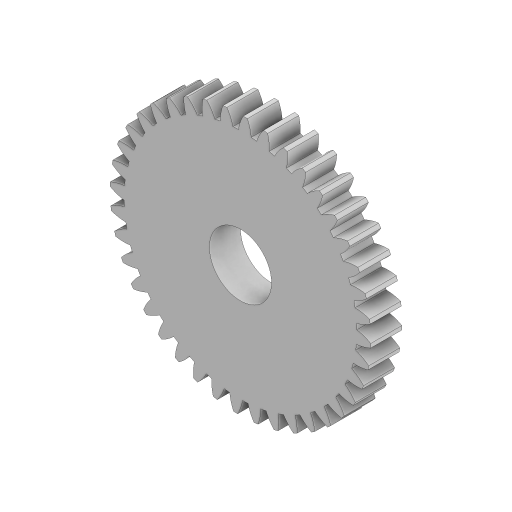
# Autodesk Inventor part: ENGRANAJE PARA RODILLO CONDUCIDO
Saved by Autodesk Inventor 2024 (Build 280153000, 153)
## iProperties
Created: 2024-06-28
Part Number: ENGRANAJE PARA RODILLO CONDUCIDO
Material: Generic
Document SubType Name: Modeling
Designer: Jhuliams
Density: 1 g/cm^3
Appearance: Default
Author: Jhuliams
Autodesk Inventor part; units mm, degrees
ref_plane "YZ Plane" through (0, 0, 0) normal (1, 0, 0) x (0, 1, 0)
ref_plane "XZ Plane" through (0, 0, 0) normal (0, 1, 0) x (-1, 0, 0)
ref_plane "XY Plane" through (0, 0, 0) normal (0, 0, 1) x (1, 0, 0)
sketch "Sketch1" plane through (0, 0, 0) normal (0, 0, 1) x (1, 0, 0)
  arc A0 (41.9411, -2.2239) -> (41.9901, -0.9106) centre (0, 0) ccw
  circle A1 centre (0, 0) radius 37.5
  line L0 (0, 0) -> (54.0602, 0) construction
  line L1 (0, 0) -> (50, 0) construction
  arc A2 (41.9901, -0.9106) -> (37.4943, 0.6513) centre (35.3209, -12.8558) ccw
  arc A3 (37.3413, -3.4461) -> (41.9411, -2.2239) centre (36.1814, 10.1854) ccw
  arc A4 (41.7726, 4.3645) -> (41.6156, 5.6693) centre (0, 0) ccw
  arc A5 (41.6156, 5.6693) -> (36.9308, 6.5087) centre (36.8971, -7.1721) ccw
  arc A6 (37.4207, 2.4377) -> (41.7726, 4.3645) centre (34.1426, 15.72) ccw
  arc A7 (40.5756, 10.8455) -> (40.2164, 12.1096) centre (0, 0) ccw
  arc A8 (40.2164, 12.1096) -> (35.458, 12.2058) centre (37.5648, -1.3118) ccw
  arc A9 (36.5786, 8.2616) -> (40.5756, 10.8455) centre (31.2631, 20.8676) ccw
  arc A10 (38.3794, 17.0593) -> (37.8269, 18.2517) centre (0, 0) ccw
  arc A11 (37.8269, 18.2517) -> (33.112, 17.6024) centre (37.3075, 4.5808) ccw
  arc A12 (34.8359, 13.8821) -> (38.3794, 17.0593) centre (27.6138, 25.5013) ccw
  arc A13 (35.2382, 22.8532) -> (34.506, 23.9445) centre (0, 0) ccw
  arc A14 (34.506, 23.9445) -> (29.9507, 22.5655) centre (36.1316, 10.3606) ccw
  arc A15 (32.2354, 19.1607) -> (35.2382, 22.8532) centre (23.2845, 29.507) ccw
  arc A16 (31.2294, 28.0843) -> (30.3354, 29.0476) centre (0, 0) ccw
  arc A17 (30.3354, 29.0476) -> (26.052, 26.973) centre (34.066, 15.8853) ccw
  arc A18 (28.8411, 23.9675) -> (31.2294, 28.0843) centre (18.3819, 32.7863) ccw
  arc A19 (26.4515, 32.6239) -> (25.4179, 33.4355) centre (0, 0) ccw
  arc A20 (25.4179, 33.4355) -> (21.5117, 30.7164) centre (31.1616, 21.0188) ccw
  arc A21 (24.7367, 28.1842) -> (26.4515, 32.6239) centre (13.0267, 35.2582) ccw
  arc A22 (21.0224, 36.3602) -> (19.8745, 37.0001) centre (0, 0) ccw
  arc A23 (19.8745, 37.0001) -> (16.4418, 33.7034) centre (27.4899, 25.6348) ccw
  arc A24 (20.0231, 31.7068) -> (21.0224, 36.3602) centre (7.3508, 36.8619) ccw
  arc A25 (15.0756, 39.2011) -> (13.8417, 39.6536) centre (0, 0) ccw
  arc A26 (13.8417, 39.6536) -> (10.967, 35.8605) centre (23.1413, 29.6195) ccw
  arc A27 (14.8166, 34.4488) -> (15.0756, 39.2011) centre (1.4938, 37.558) ccw
  arc A28 (8.7575, 41.0768) -> (7.4681, 41.3307) centre (0, 0) ccw
  arc A29 (7.4681, 41.3307) -> (5.2221, 37.1346) centre (18.2229, 32.8749) ccw
  arc A30 (9.2452, 36.3425) -> (8.7575, 41.0768) centre (-4.4, 37.3293) ccw
  arc A31 (2.2239, 41.9411) -> (0.9106, 41.9901) centre (0, 0) ccw
  arc A32 (0.9106, 41.9901) -> (-0.6513, 37.4943) centre (12.8558, 35.3209) ccw
  arc A33 (3.4461, 37.3413) -> (2.2239, 41.9411) centre (-10.1854, 36.1814) ccw
  arc A34 (-4.3645, 41.7726) -> (-5.6693, 41.6156) centre (0, 0) ccw
  arc A35 (-5.6693, 41.6156) -> (-6.5087, 36.9308) centre (7.1721, 36.8971) ccw
  arc A36 (-2.4377, 37.4207) -> (-4.3645, 41.7726) centre (-15.72, 34.1426) ccw
  arc A37 (-10.8455, 40.5756) -> (-12.1096, 40.2164) centre (0, 0) ccw
  arc A38 (-12.1096, 40.2164) -> (-12.2058, 35.458) centre (1.3118, 37.5648) ccw
  arc A39 (-8.2616, 36.5786) -> (-10.8455, 40.5756) centre (-20.8676, 31.2631) ccw
  arc A40 (-17.0593, 38.3794) -> (-18.2517, 37.8269) centre (0, 0) ccw
  arc A41 (-18.2517, 37.8269) -> (-17.6024, 33.112) centre (-4.5808, 37.3075) ccw
  arc A42 (-13.8821, 34.8359) -> (-17.0593, 38.3794) centre (-25.5013, 27.6138) ccw
  arc A43 (-22.8532, 35.2382) -> (-23.9445, 34.506) centre (0, 0) ccw
  arc A44 (-23.9445, 34.506) -> (-22.5655, 29.9507) centre (-10.3606, 36.1316) ccw
  arc A45 (-19.1607, 32.2354) -> (-22.8532, 35.2382) centre (-29.507, 23.2845) ccw
  arc A46 (-28.0843, 31.2294) -> (-29.0476, 30.3354) centre (0, 0) ccw
  arc A47 (-29.0476, 30.3354) -> (-26.973, 26.052) centre (-15.8853, 34.066) ccw
  arc A48 (-23.9675, 28.8411) -> (-28.0843, 31.2294) centre (-32.7863, 18.3819) ccw
  arc A49 (-32.6239, 26.4515) -> (-33.4355, 25.4179) centre (0, 0) ccw
  arc A50 (-33.4355, 25.4179) -> (-30.7164, 21.5117) centre (-21.0188, 31.1616) ccw
  arc A51 (-28.1842, 24.7367) -> (-32.6239, 26.4515) centre (-35.2582, 13.0267) ccw
  arc A52 (-36.3602, 21.0224) -> (-37.0001, 19.8745) centre (0, 0) ccw
  arc A53 (-37.0001, 19.8745) -> (-33.7034, 16.4418) centre (-25.6348, 27.4899) ccw
  arc A54 (-31.7068, 20.0231) -> (-36.3602, 21.0224) centre (-36.8619, 7.3508) ccw
  arc A55 (-39.2011, 15.0756) -> (-39.6536, 13.8417) centre (0, 0) ccw
  arc A56 (-39.6536, 13.8417) -> (-35.8605, 10.967) centre (-29.6195, 23.1413) ccw
  arc A57 (-34.4488, 14.8166) -> (-39.2011, 15.0756) centre (-37.558, 1.4938) ccw
  arc A58 (-41.0768, 8.7575) -> (-41.3307, 7.4681) centre (0, 0) ccw
  arc A59 (-41.3307, 7.4681) -> (-37.1346, 5.2221) centre (-32.8749, 18.2229) ccw
  arc A60 (-36.3425, 9.2452) -> (-41.0768, 8.7575) centre (-37.3293, -4.4) ccw
  arc A61 (-41.9411, 2.2239) -> (-41.9901, 0.9106) centre (0, 0) ccw
  arc A62 (-41.9901, 0.9106) -> (-37.4943, -0.6513) centre (-35.3209, 12.8558) ccw
  arc A63 (-37.3413, 3.4461) -> (-41.9411, 2.2239) centre (-36.1814, -10.1854) ccw
  arc A64 (-41.7726, -4.3645) -> (-41.6156, -5.6693) centre (0, 0) ccw
  arc A65 (-41.6156, -5.6693) -> (-36.9308, -6.5087) centre (-36.8971, 7.1721) ccw
  arc A66 (-37.4207, -2.4377) -> (-41.7726, -4.3645) centre (-34.1426, -15.72) ccw
  arc A67 (-40.5756, -10.8455) -> (-40.2164, -12.1096) centre (0, 0) ccw
  arc A68 (-40.2164, -12.1096) -> (-35.458, -12.2058) centre (-37.5648, 1.3118) ccw
  arc A69 (-36.5786, -8.2616) -> (-40.5756, -10.8455) centre (-31.2631, -20.8676) ccw
  arc A70 (-38.3794, -17.0593) -> (-37.8269, -18.2517) centre (0, 0) ccw
  arc A71 (-37.8269, -18.2517) -> (-33.112, -17.6024) centre (-37.3075, -4.5808) ccw
  arc A72 (-34.8359, -13.8821) -> (-38.3794, -17.0593) centre (-27.6138, -25.5013) ccw
  arc A73 (-35.2382, -22.8532) -> (-34.506, -23.9445) centre (0, 0) ccw
  arc A74 (-34.506, -23.9445) -> (-29.9507, -22.5655) centre (-36.1316, -10.3606) ccw
  arc A75 (-32.2354, -19.1607) -> (-35.2382, -22.8532) centre (-23.2845, -29.507) ccw
  arc A76 (-31.2294, -28.0843) -> (-30.3354, -29.0476) centre (0, 0) ccw
  arc A77 (-30.3354, -29.0476) -> (-26.052, -26.973) centre (-34.066, -15.8853) ccw
  arc A78 (-28.8411, -23.9675) -> (-31.2294, -28.0843) centre (-18.3819, -32.7863) ccw
  arc A79 (-26.4515, -32.6239) -> (-25.4179, -33.4355) centre (0, 0) ccw
  arc A80 (-25.4179, -33.4355) -> (-21.5117, -30.7164) centre (-31.1616, -21.0188) ccw
  arc A81 (-24.7367, -28.1842) -> (-26.4515, -32.6239) centre (-13.0267, -35.2582) ccw
  arc A82 (-21.0224, -36.3602) -> (-19.8745, -37.0001) centre (0, 0) ccw
  arc A83 (-19.8745, -37.0001) -> (-16.4418, -33.7034) centre (-27.4899, -25.6348) ccw
  arc A84 (-20.0231, -31.7068) -> (-21.0224, -36.3602) centre (-7.3508, -36.8619) ccw
  arc A85 (-15.0756, -39.2011) -> (-13.8417, -39.6536) centre (0, 0) ccw
  arc A86 (-13.8417, -39.6536) -> (-10.967, -35.8605) centre (-23.1413, -29.6195) ccw
  arc A87 (-14.8166, -34.4488) -> (-15.0756, -39.2011) centre (-1.4938, -37.558) ccw
  arc A88 (-8.7575, -41.0768) -> (-7.4681, -41.3307) centre (0, 0) ccw
  arc A89 (-7.4681, -41.3307) -> (-5.2221, -37.1346) centre (-18.2229, -32.8749) ccw
  arc A90 (-9.2452, -36.3425) -> (-8.7575, -41.0768) centre (4.4, -37.3293) ccw
  arc A91 (-2.2239, -41.9411) -> (-0.9106, -41.9901) centre (0, 0) ccw
  arc A92 (-0.9106, -41.9901) -> (0.6513, -37.4943) centre (-12.8558, -35.3209) ccw
  arc A93 (-3.4461, -37.3413) -> (-2.2239, -41.9411) centre (10.1854, -36.1814) ccw
  arc A94 (4.3645, -41.7726) -> (5.6693, -41.6156) centre (0, 0) ccw
  arc A95 (5.6693, -41.6156) -> (6.5087, -36.9308) centre (-7.1721, -36.8971) ccw
  arc A96 (2.4377, -37.4207) -> (4.3645, -41.7726) centre (15.72, -34.1426) ccw
  arc A97 (10.8455, -40.5756) -> (12.1096, -40.2164) centre (0, 0) ccw
  arc A98 (12.1096, -40.2164) -> (12.2058, -35.458) centre (-1.3118, -37.5648) ccw
  arc A99 (8.2616, -36.5786) -> (10.8455, -40.5756) centre (20.8676, -31.2631) ccw
  arc A100 (17.0593, -38.3794) -> (18.2517, -37.8269) centre (0, 0) ccw
  arc A101 (18.2517, -37.8269) -> (17.6024, -33.112) centre (4.5808, -37.3075) ccw
  arc A102 (13.8821, -34.8359) -> (17.0593, -38.3794) centre (25.5013, -27.6138) ccw
  arc A103 (22.8532, -35.2382) -> (23.9445, -34.506) centre (0, 0) ccw
  arc A104 (23.9445, -34.506) -> (22.5655, -29.9507) centre (10.3606, -36.1316) ccw
  arc A105 (19.1607, -32.2354) -> (22.8532, -35.2382) centre (29.507, -23.2845) ccw
  arc A106 (28.0843, -31.2294) -> (29.0476, -30.3354) centre (0, 0) ccw
  arc A107 (29.0476, -30.3354) -> (26.973, -26.052) centre (15.8853, -34.066) ccw
  arc A108 (23.9675, -28.8411) -> (28.0843, -31.2294) centre (32.7863, -18.3819) ccw
  arc A109 (32.6239, -26.4515) -> (33.4355, -25.4179) centre (0, 0) ccw
  arc A110 (33.4355, -25.4179) -> (30.7164, -21.5117) centre (21.0188, -31.1616) ccw
  arc A111 (28.1842, -24.7367) -> (32.6239, -26.4515) centre (35.2582, -13.0267) ccw
  arc A112 (36.3602, -21.0224) -> (37.0001, -19.8745) centre (0, 0) ccw
  arc A113 (37.0001, -19.8745) -> (33.7034, -16.4418) centre (25.6348, -27.4899) ccw
  arc A114 (31.7068, -20.0231) -> (36.3602, -21.0224) centre (36.8619, -7.3508) ccw
  arc A115 (39.2011, -15.0756) -> (39.6536, -13.8417) centre (0, 0) ccw
  arc A116 (39.6536, -13.8417) -> (35.8605, -10.967) centre (29.6195, -23.1413) ccw
  arc A117 (34.4488, -14.8166) -> (39.2011, -15.0756) centre (37.558, -1.4938) ccw
  arc A118 (41.0768, -8.7575) -> (41.3307, -7.4681) centre (0, 0) ccw
  arc A119 (41.3307, -7.4681) -> (37.1346, -5.2221) centre (32.8749, -18.2229) ccw
  arc A120 (36.3425, -9.2452) -> (41.0768, -8.7575) centre (37.3293, 4.4) ccw
  point P0 (37.4207, 2.4377)
  point P1 (36.9308, 6.5087)
  point P2 (33.112, 17.6024)
  point P3 (32.2354, 19.1607)
  point P4 (29.9507, 22.5655)
  point P5 (28.8411, 23.9675)
  point P6 (26.052, 26.973)
  point P7 (20.0231, 31.7068)
  point P8 (16.4418, 33.7034)
  point P9 (10.967, 35.8605)
  point P10 (9.2452, 36.3425)
  point P11 (5.2221, 37.1346)
  point P12 (3.4461, 37.3413)
  point P13 (-0.6513, 37.4943)
  point P14 (-2.4377, 37.4207)
  point P15 (-6.5087, 36.9308)
  point P16 (-12.2058, 35.458)
  point P17 (-17.6024, 33.112)
  point P18 (-23.9675, 28.8411)
  point P19 (-26.973, 26.052)
  point P20 (-31.7068, 20.0231)
  point P21 (-35.8605, 10.967)
  point P22 (-37.1346, 5.2221)
  point P23 (-37.3413, 3.4461)
  point P24 (-37.4943, -0.6513)
  point P25 (-37.4207, -2.4377)
  point P26 (-36.9308, -6.5087)
  point P27 (-36.5786, -8.2616)
  point P28 (-35.458, -12.2058)
  point P29 (-33.112, -17.6024)
  point P30 (-26.052, -26.973)
  point P31 (-16.4418, -33.7034)
  point P32 (-10.967, -35.8605)
  point P33 (-9.2452, -36.3425)
  point P34 (-5.2221, -37.1346)
  point P35 (-3.4461, -37.3413)
  point P36 (0.6513, -37.4943)
  point P37 (2.4377, -37.4207)
  point P38 (6.5087, -36.9308)
  point P39 (12.2058, -35.458)
  point P40 (13.8821, -34.8359)
  point P41 (17.6024, -33.112)
  point P42 (19.1607, -32.2354)
  point P43 (22.5655, -29.9507)
  point P44 (26.973, -26.052)
  point P45 (28.1842, -24.7367)
  point P46 (30.7164, -21.5117)
  point P47 (33.7034, -16.4418)
  point P48 (34.4488, -14.8166)
  point P49 (35.8605, -10.967)
  point P50 (36.3425, -9.2452)
  point P51 (37.1346, -5.2221)
  point P52 (37.3413, -3.4461)
  dimension "d2" = 75
  dimension "d1" = 84
  dimension "d8" = 360
  constraints: 240 point on circle, 120 centre point, 4 end point, 2 horizontal, 1 coincident, 403 other
  measures "d1" diameter of A0
extrude "Extrusion1" add sketch "Sketch1" along normal blind 10
sketch "Sketch2" plane through (0, 0, 10) normal (0, 0, 1) x (1, 0, 0)
  circle A0 centre (0, 0) radius 10
  dimension "d12" = 20
  constraints: 1 centre point, 1 coincident
  measures "d12" diameter of A0
extrude "Extrusion2" cut sketch "Sketch2" against normal blind 20
body "Solid1"
